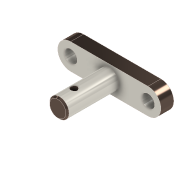
# Autodesk Inventor part: Crank
Saved by Autodesk Inventor 2022.2 (Build 262287010, 287A)
## iProperties
Created: 2022-12-29
Part Number: Crank
Material: Steel
Document SubType Name: Modeling
Designer: User
Mass: 10.2058 g
Surface Area: 11.5327 cm^2
Volume: 1.3001 cm^3
Density: 7.85 g/cm^3
Appearance: Gunmetal - Antique Polished
Author: User
Autodesk Inventor part; units mm, degrees
ref_plane "XZ Plane" through (0, 0, 0) normal (0, 1, 0) x (-1, 0, 0)
ref_plane "XY Plane" through (0, 0, 0) normal (0, 0, 1) x (1, 0, 0)
sketch "Sketch1" plane through (0, 0, 0) normal (0, 0, 1) x (1, 0, 0)
  line L0 (-12, 0) -> (12, 0) construction
  line L1 (-12, -4) -> (12, -4)
  line L2 (12, 4) -> (-12, 4)
  arc A0 (-12, 4) -> (-12, -4) centre (-12, 0) ccw
  arc A1 (12, -4) -> (12, 4) centre (12, 0) ccw
  point P0 (0, 0)
  dimension "d0" = 24
  dimension "d1" = 4
  constraints: 8 end point, 4 point on circle, 4 tangent, 2 centre point, 1 horizontal, 1 midpoint, 1 parallel
  measures "d0" distance of L2.start L2.end
  measures "d1" radius of A1
extrude "Extrusion1" add sketch "Sketch1" along normal blind 4
sketch "Sketch2" plane through (0, 0, 4) normal (0, 0, 1) x (1, 0, 0)
  circle A0 centre (0, 0) radius 3
  dimension "d4" = 6
  constraints: 1 centre point, 1 coincident
  measures "d4" diameter of A0
extrude "Extrusion2" add sketch "Sketch2" along normal blind 16
chamfer "Chamfer1" distance 0.5 angle 45 1 edges at (-3, 0, 20)
sketch "Sketch3" plane through (0, 0, 4) normal (0, 0, 1) x (1, 0, 0)
  arc A0 (12, -4) -> (12, 4) centre (12, 0) ccw projected
  arc A1 (-12, 4) -> (-12, -4) centre (-12, 0) ccw projected
hole "Hole1" at (-12, 0, 4) at (12, 0, 4) direction (0, 0, -1) diameter 4 end through all
ref_plane "Work Plane1" through (0, 0, 15) normal (0, 0, 1) x (1, 0, 0)
hole "Hole2" at (0, 3, 15) direction (0, -1, 0) diameter 2 end through all
body "Solid1"
